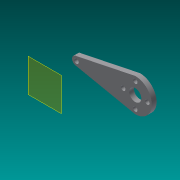
# Autodesk Inventor part: headtilt-teardrop
Saved by Autodesk Inventor 2013 SP2 (Build 170200200, 200)
## iProperties
Created: 2014-11-25
Part Number: headtilt-teardrop
Material: Generic
Document SubType Name: Sheet Metal
Designer: Master
Density: 1 g/cm^3
Sheet Metal Rule: Default
Author: Master
Autodesk Inventor part; units mm, degrees
ref_plane "YZ Plane" through (0, 0, 0) normal (1, 0, 0) x (0, 1, 0)
ref_plane "XZ Plane" through (0, 0, 0) normal (0, 1, 0) x (-1, 0, 0)
ref_plane "XY Plane" through (0, 0, 0) normal (0, 0, 1) x (1, 0, 0)
sketch "Sketch1" plane through (0, 0, 0) normal (0, 0, 1) x (1, 0, 0)
  line L0 (53.6991, 27.6003) -> (52.1809, 27.6003)
  arc A0 (53.6991, 27.1003) -> (53.6991, 27.6003) centre (55.1781, 27.3503) ccw
  line L1 (52.1809, 27.1003) -> (53.6991, 27.1003)
  arc A1 (52.1809, 27.1003) -> (52.1809, 27.6003) centre (63.1781, 27.3503) ccw
  circle A2 centre (63.1781, 35.3503) radius 1.5
  circle A3 centre (63.1781, 19.3503) radius 1.5
  circle A4 centre (71.1781, 27.3503) radius 1.5
  circle A5 centre (63.1781, 27.3503) radius 4
  circle A6 centre (24.1779, 27.3503) radius 1.4986
  arc A7 (24.1777, 30.2419) -> (24.1781, 24.4588) centre (24.1779, 27.3503) ccw
  line L2 (24.1777, 30.2419) -> (63.1781, 38.3503)
  line L3 (24.1781, 24.4588) -> (63.1794, 16.3503)
  arc A8 (63.1794, 16.3503) -> (63.1781, 38.3503) centre (63.1781, 27.3503) ccw
  circle A9 centre (63.1781, 35.3503) radius 1.5
  arc A10 (53.6991, 27.1003) -> (53.6991, 27.6003) centre (55.1781, 27.3503) ccw
  circle A11 centre (63.1781, 19.3503) radius 1.5
  circle A12 centre (71.1781, 27.3503) radius 1.5
  circle A13 centre (55.1781, 27.3503) radius 1.5
  circle A14 centre (63.1781, 35.3503) radius 1.5
  circle A15 centre (63.1781, 19.3503) radius 1.5
  circle A16 centre (71.1781, 27.3503) radius 1.5
  circle A17 centre (63.1781, 27.3503) radius 1.75
  circle A18 centre (63.1781, 27.3503) radius 1.75
  point P0 (0, 0)
  dimension "d1" = 2.9972
  measures "d1" diameter of A6
ref_plane "Work Plane2" through (0, 0, 0) normal (0, 0, 1) x (1, 0, 0)
extrude "Plate1" add sketch "Sketch1" along normal blind 3.175 contours A13 L1 A1 L3 A7 L2 L0 | L0 A1 L2 L3 L1 A0
equation "\"BendRadius\" = Thickness"
equation "\"BendReliefWidth\" = Thickness"
equation "\"BendReliefDepth\" = 0.5 * Thickness"
equation "\"CornerReliefSize\" = 4 * Thickness"
equation "\"MinimumRemnant\" = 2 * Thickness"
equation "\"TransitionRadius\" = BendRadius"
equation "\"JacobiRadiusSize\" = BendRadius"
equation "\"GapSize\" = Thickness"
equation "\"d2\" = BendRadius"
equation "\"Thickness\" = 3.175"
body "Solid1"
